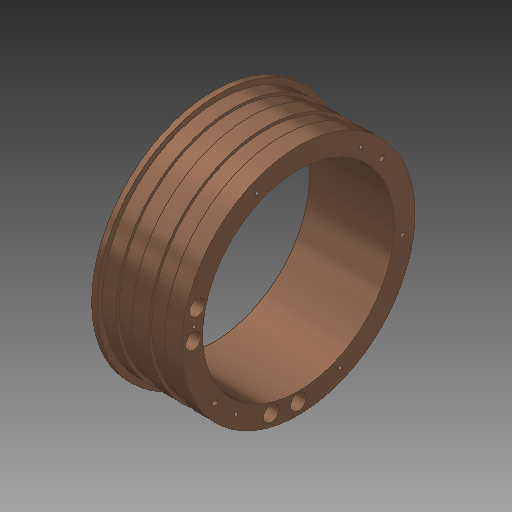
# Autodesk Inventor part: 1131_Inner RU Body_V1
Saved by Autodesk Inventor 2020 (Build 240168000, 168)
## iProperties
Created: 2017-08-07
Part Number: 1131_Inner RU Body_V1
Material: Bronze
Document SubType Name: Modeling
Designer: MPI
Density: 8.47 g/cm^3
Appearance: Brass - Satin
Mass: 1997.1 g
Surface Area: 594.297 cm^2
Volume: 235.785 cm^3
Author: MPI
Autodesk Inventor part; units mm, degrees
ref_plane "YZ Plane" through (0, 0, 0) normal (1, 0, 0) x (0, 1, 0)
ref_plane "XZ Plane" through (0, 0, 0) normal (0, 1, 0) x (-1, 0, 0)
ref_plane "XY Plane" through (0, 0, 0) normal (0, 0, 1) x (1, 0, 0)
sketch "Sketch1" plane through (0, 0, 0) normal (0, 0, 1) x (1, 0, 0)
  line L0 (-22.2356, 0) -> (22.2356, 0) construction
  line L1 (0, 69.723) -> (47.625, 69.723)
  line L2 (0, 69.723) -> (0, 72.898)
  line L3 (0, 72.898) -> (-3.175, 72.898)
  line L4 (-3.175, 72.898) -> (-3.175, 57.404)
  line L5 (-3.175, 57.404) -> (47.625, 57.404)
  line L6 (47.625, 57.404) -> (47.625, 69.723)
  line L7 (8.4328, 69.723) -> (17.9578, 69.723)
  line L8 (17.9578, 69.723) -> (17.9578, 68.1355)
  line L9 (17.9578, 68.1355) -> (8.4328, 68.1355)
  line L10 (37.465, 69.723) -> (27.94, 69.723)
  line L11 (27.94, 69.723) -> (27.94, 68.1355)
  line L12 (27.94, 68.1355) -> (37.465, 68.1355)
  line L13 (37.465, 68.1355) -> (37.465, 69.723)
  line L14 (8.4328, 69.723) -> (8.4328, 68.1355)
  point P0 (0, 0)
  point P1 (0, 0)
  dimension "d1" = 139.446
  dimension "d2" = 69.723
  dimension "d3" = 3.175
  dimension "d4" = 3.175
  dimension "d5" = 114.808
  dimension "d6" = 1.5875
  dimension "d7" = 9.525
  dimension "d12" = 50.8
  dimension "d15" = 9.525
  dimension "d16" = 19.685
  dimension "d17" = 11.6078
  dimension "d18" = 1.5875
  constraints: 30 end point, 7 perpendicular, 4 point on line, 3 parallel, 2 horizontal, 1 coincident, 1 midpoint, 1 vertical, 1 vertical alignment
  measures "d1" diameter of L1 L0
  measures "d2" distance from line of point (0, 0) L1
  measures "d3" distance of L1.start L2.end
  measures "d4" distance of L2.end L3.end
  measures "d5" diameter of L5 L0
  measures "d6" distance of L7.end L8.end
  measures "d7" distance of L10.start L10.end
  measures "d12" distance between parallel lines of L6 L4
  measures "d15" distance of L7.start L7.end
  measures "d16" distance between parallel lines of L6 L11
  measures "d17" distance between parallel lines of L14 L4
  measures "d18" distance between parallel lines of L1 L12
revolve "Revolution1" add sketch "Sketch1" angle 360 about axis through (-22.2356, 0, 0) along (1, 0, 0) contours L1 L14 L9 L8 L11 L12 L13 L6 L5 L4 L3 L2
sketch "Sketch2" plane through (47.625, 0, 0) normal (1, 0, 0) x (0, 0, -1)
  circle A0 centre (0, 0) radius 57.404 projected
  circle A1 centre (0, 0) radius 68.1355 projected
  circle A2 centre (0, 0) radius 68.1355 projected
  line L0 (-68.1355, 0) -> (-57.404, 0)
  circle A3 centre (-62.7698, 0) radius 4.7625
  point P0 (-58.0072, 0)
  dimension "d19" = 9.525
  constraints: 2 end point, 2 horizontal alignment, 2 point on circle, 1 horizontal, 1 midpoint, 1 point on line, 3 other
extrude "Extrusion1" cut sketch "Sketch2" against normal blind 7.62 contours A3 L0 | L0 A3
sketch "Sketch3" plane through (40.005, 0, 62.7698) normal (1, 0, 0) x (0, 0, -1)
  circle A0 centre (0, 0) radius 4.7625 projected
  circle A1 centre (0, 0) radius 3.175
  point P0 (62.7698, 0)
  dimension "d22" = 6.35
  constraints: 1 centre point, 1 coincident
  measures "d22" diameter of A1
extrude "Extrusion2" cut sketch "Sketch3" against normal up to surface (12.065 mm away) contours A1
pattern_circular "Circular Pattern1" count 2 over 15 about axis through (22.225, 0, 0) along (-1, 0, 0) of "Extrusion2", "Extrusion1"
pattern_circular "Circular Pattern2" count 2 over 90 about axis through (22.225, 0, 0) along (1, 0, 0) of "Extrusion2", "Extrusion1", "Circular Pattern1"
sketch "Sketch4" plane through (27.94, -60.6309, 16.246) normal (1, 0, 0) x (0, 0, -1)
  circle A0 centre (0, 0) radius 3.175 projected
  circle A1 centre (16.246, -2.1388) radius 3.175 projected
  point P0 (16.246, 60.6309)
extrude "Extrusion3" cut sketch "Sketch4" against normal up to surface (19.5072 mm away)
sketch "Sketch5" plane through (47.625, 0, 0) normal (1, 0, 0) x (0, 0, -1)
  circle A0 centre (-16.246, -60.6309) radius 4.7625 construction
  circle A1 centre (0, -62.7698) radius 4.7625 construction
  circle A2 centre (-60.6309, 16.246) radius 4.7625 construction
  circle A3 centre (-62.7698, 0) radius 4.7625 construction
  circle A4 centre (0, 0) radius 69.723 construction
  circle A5 centre (0, 0) radius 57.404 construction
  circle A6 centre (0, 0) radius 69.723 construction
  circle A7 centre (-16.246, -60.6309) radius 3.175 construction
  line L0 (-16.246, -60.6309) -> (0, 0) construction
  line L1 (0, 0) -> (-62.7698, 0) construction
  circle A8 centre (-49.9749, -38.3471) radius 1.651
  circle A9 centre (49.9749, 38.3471) radius 1.6475
  line L2 (-55.315, -42.4447) -> (-45.5417, -34.9453)
  line L3 (45.5417, 34.9453) -> (55.315, 42.4447)
  point P0 (0, 0)
  point P1 (0, 0)
  dimension "d33" = 75
  dimension "d35" = 3.302
  dimension "d36" = 5.588
  dimension "d38" = 5.588
  constraints: 8 end point, 3 point on circle, 2 centre point, 2 point on line, 1 coincident, 1 horizontal, 2 other
  measures "d33" angle of L1 L0
  measures "d35" diameter of A8
  measures "d36" distance of A8.centre L2.end
  measures "d38" distance of A9.centre L3.start
extrude "Extrusion4" cut sketch "Sketch5" against normal blind 25.4
sketch "Sketch6" plane through (47.625, 0, 0) normal (1, 0, 0) x (0, 0, -1)
  circle A0 centre (49.9749, 38.3471) radius 1.6475 construction
  circle A1 centre (-49.9749, -38.3471) radius 1.651 construction
  circle A2 centre (-16.246, -60.6309) radius 4.7625 construction
  circle A3 centre (0, -62.7698) radius 4.7625 construction
  circle A4 centre (-60.6309, 16.246) radius 4.7625 construction
  circle A5 centre (-62.7698, 0) radius 4.7625 construction
  circle A6 centre (0, 0) radius 69.723 construction
  circle A7 centre (0, 0) radius 57.404 construction
  circle A8 centre (0, 0) radius 62.7698 construction
  line L0 (0, 0) -> (0, -62.7698) construction
  circle A9 centre (0, -62.7698) radius 3.175 projected
  circle A10 centre (0, -62.7698) radius 25.4 construction
  point P0 (0, 0)
  point P1 (24.8747, -57.6307)
  dimension "d41" = 50.8
  constraints: 2 coincident, 2 end point, 2 point on circle, 1 centre point, 1 vertical, 3 other
hole "Hole1" at (47.625, -57.6307, -24.8747) direction (-1, 0, 0) diameter 2.159 depth 8.8646 tip angle 118
pattern_circular "Circular Pattern3" count 6 over 360 about axis through (22.225, 0, 0) along (1, 0, 0) of "Hole1"
equation "\"d18\" = d6"
equation "\"d38\" = d36"
equation "\"d34\" = 0.5 * d33"
body "Solid1"
